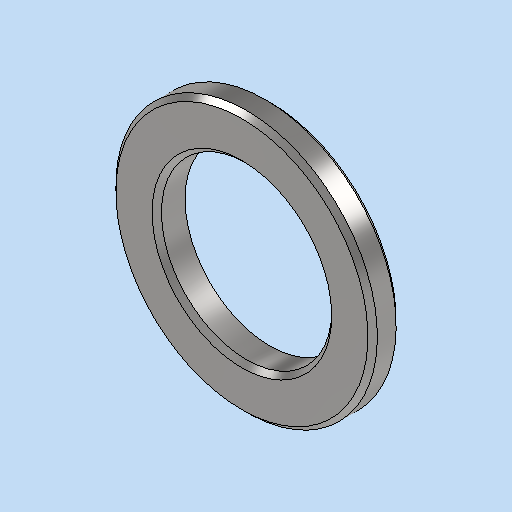
# Autodesk Inventor part: boron-target-grooved-spacer
Saved by Autodesk Inventor 2025 (Build 290162000, 162)
## iProperties
Created: 2024-12-16
Part Number: boron-target-grooved-spacer
Material: Stainless Steel
Document SubType Name: Modeling
Designer: kuzmin
Density: 8 g/cm^3
Appearance: Semi-Polished
Author: kuzmin
Autodesk Inventor part; units mm, degrees
ref_plane "YZ Plane" through (0, 0, 0) normal (1, 0, 0) x (0, 1, 0)
ref_plane "XZ Plane" through (0, 0, 0) normal (0, 1, 0) x (-1, 0, 0)
ref_plane "XY Plane" through (0, 0, 0) normal (0, 0, 1) x (1, 0, 0)
sketch "Sketch1" plane through (0, 0, 0) normal (1, 0, 0) x (0, 1, 0)
  line L0 (9.05, 1.5) -> (13.9, 1.5)
  line L1 (13.9, 1.5) -> (13.9, -1.5)
  line L2 (13.9, -1.5) -> (9.05, -1.5)
  line L3 (9.05, -1.5) -> (9.05, 1.5)
  line L4 (0, 0) -> (0, 7.1072) construction
  point P0 (9.05, 0)
  dimension "d0" = 27.8
  dimension "d1" = 18.1
  dimension "d2" = 3
  constraints: 10 end point, 2 parallel, 1 horizontal, 1 horizontal alignment, 1 midpoint, 1 perpendicular, 1 vertical
  measures "d0" diameter of L1 L4
  measures "d1" diameter of L3 L4
  measures "d2" distance of L0.end L1.end
revolve "Revolution1" add sketch "Sketch1" angle 360 about axis through (0, 0, 0) along (0, 0, 1)
chamfer "Chamfer1" distance 0.5 angle 45 3 edges at (0, -13.9, -1.5) (0, -13.9, 1.5) (0, -9.05, 1.5)
body "Solid1"
